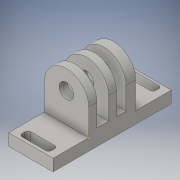
# Autodesk Inventor part: gopro_drone
Saved by Autodesk Inventor 2016 (Build 200138000, 138)
## iProperties
Created: 2015-08-22
Part Number: gopro_drone
Material: Generic
Document SubType Name: Modeling
Designer: Tyler
Density: 1 g/cm^3
Appearance: Default
Author: Tyler
Autodesk Inventor part; units mm, degrees
ref_plane "YZ Plane" through (0, 0, 0) normal (1, 0, 0) x (0, 1, 0)
ref_plane "XZ Plane" through (0, 0, 0) normal (0, 1, 0) x (-1, 0, 0)
ref_plane "XY Plane" through (0, 0, 0) normal (0, 0, 1) x (1, 0, 0)
sketch "Sketch4" plane through (0, 0, 0) normal (0, 0, 1) x (1, 0, 0)
  line L0 (-10.5, 0) -> (10.5, 0) projected
  line L1 (0, -3.3) -> (0, 19.8) projected
  line L2 (-7.5, 0) -> (7.5, 0)
  line L3 (7.5, 0) -> (7.5, 16.5)
  line L4 (7.5, 16.5) -> (-7.5, 16.5)
  line L5 (-7.5, 16.5) -> (-7.5, 0)
  circle A0 centre (0, 10) radius 2.5
  point P0 (0, 0)
  dimension "d0" = 7.5
  dimension "d1" = 7.5
  dimension "d2" = 16.5
  dimension "d3" = 5
  dimension "d4" = 6.5
  constraints: 8 end point, 2 parallel, 2 point on line, 1 centre point, 1 horizontal, 1 perpendicular
  measures "d0" distance between parallel lines of L1 L5
  measures "d1" distance between parallel lines of L1 L3
  measures "d2" distance between parallel lines of L4 L0
  measures "d3" diameter of A0
  measures "d4" distance from line of L4 A0.centre
extrude "Extrusion1" add sketch "Sketch4" against normal blind 15.9 contours L5 L4 L1 A0 L0 | L1 A0 L4 L3 L0
fillet "Fillet1" radius 7.5 2 edges at (7.5, 16.5, -7.95) (-7.5, 16.5, -7.95)
sketch "Sketch6" plane through (7.5, 9, 0) normal (1, 0, 0) x (0, 0, -1)
  point P0 (0, -9)
sketch "Sketch7" plane through (7.5, 9, 0) normal (1, 0, 0) x (0, 0, -1)
  line L0 (0, 0) -> (0, 7.5) projected
  line L1 (0, 7.5) -> (3.3, 7.5)
  line L2 (3.3, 7.5) -> (3.3, -7.5)
  line L3 (3.3, -7.5) -> (0, -7.5)
  line L4 (0, -7.5) -> (0, 7.5)
  line L5 (0, 7.5) -> (15.9, 7.5) projected
  line L6 (6.3, 7.5) -> (9.6, 7.5)
  line L7 (9.6, 7.5) -> (9.6, -7.5)
  line L8 (9.6, -7.5) -> (6.3, -7.5)
  line L9 (6.3, -7.5) -> (6.3, 7.5)
  line L10 (12.6, 7.5) -> (15.9, 7.5)
  line L11 (15.9, 7.5) -> (15.9, -7.5)
  line L12 (15.9, -7.5) -> (12.6, -7.5)
  line L13 (12.6, -7.5) -> (12.6, 7.5)
  line L14 (3.3, -7.5) -> (6.3, -7.5)
  line L15 (9.6, -7.5) -> (12.6, -7.5)
  line L16 (3.3, 7.5) -> (6.3, 7.5)
  line L17 (9.6, 7.5) -> (12.6, 7.5)
  point P0 (0, -9)
  dimension "d10" = 3.3
  dimension "d11" = 15
  dimension "d12" = 3
  dimension "d13" = 3.3
  dimension "d14" = 3
  dimension "d15" = 3.3
  constraints: 32 end point, 6 parallel, 4 horizontal, 4 point on line, 3 collinear, 3 perpendicular
  measures "d10" distance between parallel lines of L2 L0
  measures "d11" distance of L1.end L2.end
  measures "d12" distance between parallel lines of L9 L2
  measures "d13" distance between parallel lines of L7 L9
  measures "d14" distance between parallel lines of L7 L13
  measures "d15" distance between parallel lines of L11 L13
sketch "Sketch8" plane through (7.5, 9, 0) normal (1, 0, 0) x (0, 0, -1)
  line L0 (0, 7.5) -> (15.9, 7.5) projected
  line L1 (2.8, 7.5) -> (6.55, 7.5)
  line L2 (6.55, 7.5) -> (6.55, -7.4999)
  line L3 (6.55, -7.4999) -> (2.8, -7.4999)
  line L4 (2.8, -7.4999) -> (2.8, 7.5)
  line L5 (9.35, 7.5) -> (13.1, 7.5)
  line L6 (13.1, 7.5) -> (13.1, -7.4999)
  line L7 (13.1, -7.4999) -> (9.35, -7.4999)
  line L8 (9.35, -7.4999) -> (9.35, 7.5)
  line L9 (0, 0) -> (0, 7.5) projected
  line L10 (15.9, 7.5) -> (15.9, 0) projected
  point P0 (0, -9)
  dimension "d42" = 2.8
  dimension "d43" = 2.8
  dimension "d44" = 14.9999
  dimension "d45" = 2.8
  dimension "d46" = 3.75
  constraints: 16 end point, 4 parallel, 3 point on line, 2 horizontal, 2 perpendicular
  measures "d42" distance between parallel lines of L4 L9
  measures "d43" distance between parallel lines of L8 L2
  measures "d44" distance of L5.end L6.end
  measures "d45" distance between parallel lines of L10 L6
  measures "d46" distance between parallel lines of L2 L4
extrude "Extrusion3" cut sketch "Sketch7" against normal through all contours L5 L13 L15 L7
extrude "Extrusion4" cut sketch "Sketch8" against normal through all contours L0 L2 L3 L4
sketch "Sketch10" plane through (-7.5, 0, 0) normal (0, -1, 0) x (1, 0, 0)
  line L0 (-3, 0) -> (18, 0) projected
  line L1 (7.5, -19.08) -> (7.5, 3.18) projected
  line L2 (15, 12.05) -> (0, 12.05)
  line L3 (0, 12.05) -> (0, -27.95)
  line L4 (0, -27.95) -> (15, -27.95)
  line L5 (15, -27.95) -> (15, 12.05)
  line L6 (11.5, 11.05) -> (3.5, 11.05)
  line L7 (2.5, 10.05) -> (2.5, 9.05)
  line L8 (3.5, 8.05) -> (11.5, 8.05)
  line L9 (12.5, 9.05) -> (12.5, 10.05)
  line L10 (15, -6.55) -> (15, -9.6) projected
  line L11 (15, -8.075) -> (0, -8.075)
  line L12 (0, -9.6) -> (0, -6.55) projected
  line L13 (11.5, -27.2) -> (3.5, -27.2)
  line L14 (2.5, -26.2) -> (2.5, -25.2)
  line L15 (3.5, -24.2) -> (11.5, -24.2)
  line L16 (12.5, -25.2) -> (12.5, -26.2)
  arc A0 (11.5, 8.05) -> (12.5, 9.05) centre (11.5, 9.05) ccw
  arc A1 (12.5, 10.05) -> (11.5, 11.05) centre (11.5, 10.05) ccw
  arc A2 (3.5, 11.05) -> (2.5, 10.05) centre (3.5, 10.05) ccw
  arc A3 (2.5, 9.05) -> (3.5, 8.05) centre (3.5, 9.05) ccw
  arc A4 (12.5, -25.2) -> (11.5, -24.2) centre (11.5, -25.2) ccw
  arc A5 (11.5, -27.2) -> (12.5, -26.2) centre (11.5, -26.2) ccw
  arc A6 (3.5, -24.2) -> (2.5, -25.2) centre (3.5, -25.2) ccw
  arc A7 (2.5, -26.2) -> (3.5, -27.2) centre (3.5, -26.2) ccw
  point P0 (7.5, 0)
  point P1 (12.5, 11.05)
  point P2 (2.5, 8.05)
  point P3 (2.5, 11.05)
  point P4 (12.5, 8.05)
  point P5 (12.5, -27.2)
  point P6 (2.5, -24.2)
  point P7 (2.5, -27.2)
  point P8 (12.5, -24.2)
  dimension "d20" = 15
  dimension "d21" = 40
  dimension "d22" = 12.05
  dimension "d23" = 7.5
  dimension "d24" = 3
  dimension "d25" = 1
  dimension "d26" = 10
  dimension "d27" = 2.5
  dimension "d28" = 8.075
  dimension "d29" = 1
  constraints: 26 end point, 16 point on circle, 16 point on line, 16 tangent, 8 centre point, 7 equal radius, 4 parallel, 4 symmetric about line, 2 horizontal, 2 midpoint, 2 perpendicular
  measures "d20" distance of L2.start L2.end
  measures "d21" distance between parallel lines of L4 L2
  measures "d22" distance between parallel lines of L0 L2
  measures "d23" distance between parallel lines of L1 L5
  measures "d24" distance between parallel lines of L8 L6
  measures "d25" distance between parallel lines of L6 L2
  measures "d26" distance between parallel lines of L7 L9
  measures "d27" distance between parallel lines of L5 L9
  measures "d28" distance between parallel lines of L0 L11
  measures "d29" radius of A0
extrude "Extrusion5" add sketch "Sketch10" along normal blind 4
sketch "Sketch12" plane through (7.5, 1.5, -12.6) normal (1, 0, 0) x (0, 0, -1)
  line L0 (-6.05, 15) -> (-3, 15) projected
  line L1 (-5.85, 15) -> (-6.05, 15)
  line L2 (-6.05, 15) -> (-6.05, 0.0001)
  line L3 (-6.05, 0.0001) -> (-5.85, 0.0001)
  line L4 (-5.85, 0.0001) -> (-5.85, 15)
  line L5 (-6.05, 7.5) -> (-6.05, 0.0001) projected
  line L6 (-3, 15) -> (-3, 7.5) projected
  line L7 (-3, 15) -> (-3.2, 15)
  line L8 (-3.2, 15) -> (-3.2, 0.0001)
  line L9 (-3.2, 0.0001) -> (-3, 0.0001)
  line L10 (-3, 0.0001) -> (-3, 15)
  line L11 (-12.6, -9.6) -> (-12.6, 19.1) projected
  line L12 (23.35, -1.5) -> (-32.65, -1.5) projected
  line L13 (-6.05, 15) -> (-3, 15) projected
  line L14 (3.3, 15) -> (3.3, 7.5) projected
  point P0 (-12.6, -1.5)
  dimension "d36" = 0.2
  dimension "d37" = 0
  dimension "d38" = 0
  dimension "d39" = 0.2
  constraints: 16 end point, 4 parallel, 2 horizontal, 2 perpendicular, 1 point on line
  measures "d36" distance of L2.end L3.end
  measures "d37" distance between parallel lines of L5 L2
  measures "d38" distance from line of L5.end L3
  measures "d39" distance between parallel lines of L8 L10
extrude "Extrusion7" cut sketch "Sketch12" against normal through all
body "Solid1"
